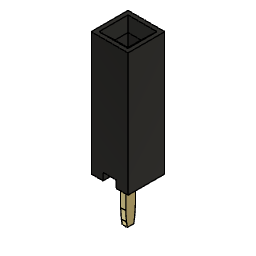
Adjustable_Header_Female (Autodesk Fusion 360 design; units mm, degrees)
Autodesk Fusion 360 part; units mm, degrees
sketch "Sketch1" plane through (0, 0, 0) normal (0, 0, 1) x (1, 0, 0)
  line L0 (1, -1) -> (-1, -1)
  line L1 (-1, -1) -> (-1, 1)
  line L2 (-1, 1) -> (1, 1)
  line L3 (1, 1) -> (1, -1)
  line L4 (1, -1) -> (-1, 1) construction
  line L5 (-1, -1) -> (1, 1) construction
  dimension "d1" = 2
  dimension "d2" = 2
  constraint horizontal L0
  constraint perpendicular L0 L1
  constraint parallel L0 L2
  constraint parallel L1 L3
  constraint coincident L4 origin
  constraint coincident L5 origin
  measures "d1" distance of L1.end L2.end
  measures "d2" distance of L0.end L1.end
extrude "Extrude1" add sketch "Sketch1" along normal blind 8.5 makes body 1
sketch "Sketch2" plane through (0, 0, 8.5) normal (0, 0, 1) x (-1, 0, 0)
  line L0 (-1, -1) -> (1, -1)
  line L1 (1, -1) -> (1, 1)
  line L2 (1, 1) -> (-1, 1)
  line L3 (-1, 1) -> (-1, -1)
  line L4 (-0.45, 0.45) -> (0.45, 0.45)
  line L5 (0.45, 0.45) -> (0.45, -0.45)
  line L6 (0.45, -0.45) -> (-0.45, -0.45)
  line L7 (-0.45, -0.45) -> (-0.45, 0.45)
  line L8 (-0.45, 0.45) -> (0.45, -0.45) construction
  line L9 (0.45, 0.45) -> (-0.45, -0.45) construction
  dimension "d5" = 0.9
  dimension "d6" = 0.9
  constraint horizontal L4
  constraint perpendicular L4 L5
  constraint parallel L4 L6
  constraint parallel L5 L7
  constraint coincident L8 origin
  constraint coincident L9 origin
  measures "d5" distance of L5.end L6.end
  measures "d6" distance of L4.end L5.end
extrude "Extrude2" cut sketch "Sketch2" against normal blind 0.5 contours L4 L5 L6 L7 bodies 1
loft "Loft1" cut profiles "Sketch2" section 1 contours L0 L1 L2 L3 | L4 L5 L6 L7 section 2 face at (0.15, -0.15, 8) on bodies 1 bodies 1
extrude "Extrude3" cut 1 faces at (0.15, -0.15, 8) along direction (0, 0, -1) through all on bodies 1 bodies 1
sketch "Sketch3" plane through (0, 0, 0) normal (0, 0, -1) x (1, 0, 0)
  line L0 (0.45, 0.45) -> (0.45, -0.45)
  line L1 (0.45, -0.45) -> (-0.45, -0.45)
  line L2 (-0.45, -0.45) -> (-0.45, 0.45)
  line L3 (-0.45, 0.45) -> (0.45, 0.45)
  line L4 (-1, -1) -> (1, -1)
  line L5 (1, -1) -> (1, 1)
  line L6 (1, 1) -> (-1, 1)
  line L7 (-1, 1) -> (-1, -1)
  line L8 (0.325, -0.175) -> (-0.325, -0.175)
  line L9 (-0.325, -0.175) -> (-0.325, 0.175)
  line L10 (-0.325, 0.175) -> (0.325, 0.175)
  line L11 (0.325, 0.175) -> (0.325, -0.175)
  line L12 (0.325, -0.175) -> (-0.325, 0.175) construction
  line L13 (-0.325, -0.175) -> (0.325, 0.175) construction
  dimension "d11" = 0.65
  dimension "d12" = 0.35
  constraint horizontal L8
  constraint perpendicular L8 L9
  constraint parallel L8 L10
  constraint parallel L9 L11
  constraint coincident L12 origin
  constraint coincident L13 origin
  measures "d11" distance of L9.end L10.end
  measures "d12" distance of L8.end L9.end
extrude "Extrude4" add sketch "Sketch3" along normal blind 3 separate body contours L8 L9 L10 L11 makes body 2
chamfer "Chamfer1" distance 0.1 distance2 0.7 2 edges at (0.325, 0, -3) (-0.325, 0, -3) measured on face at (0.1083, 0.0583, -3) measured on face at (0.1083, 0.0583, -3) on bodies 2
sketch "Sketch4" plane through (0, 0, 0) normal (0, 0, 1) x (-1, 0, 0)
  line L0 (0.325, 0.175) -> (-0.325, 0.175)
  line L1 (-0.325, 0.175) -> (-0.325, -0.175)
  line L2 (-0.325, -0.175) -> (0.325, -0.175)
  line L3 (0.325, -0.175) -> (0.325, 0.175)
  line L4 (-0.325, 0.175) -> (-0.475, 0.175)
  line L5 (-0.475, 0.175) -> (-0.475, -0.175)
  line L6 (-0.475, -0.175) -> (-0.325, -0.175)
  line L7 (-0.325, -0.175) -> (-0.325, 0.175)
  line L8 (0.325, 0.175) -> (0.475, 0.175)
  line L9 (0.475, 0.175) -> (0.475, -0.175)
  line L10 (0.475, -0.175) -> (0.325, -0.175)
  line L11 (0.325, -0.175) -> (0.325, 0.175)
  dimension "d17" = 0.15
  dimension "d18" = 0.15
  constraint horizontal L4
  constraint vertical L5
  constraint horizontal L6
  constraint vertical L7
  constraint coincident L0.end L1.start
  constraint horizontal L8
  constraint vertical L9
  constraint horizontal L10
  constraint vertical L11
  constraint coincident L0.start L3.end
  measures "d17" distance of L0.end L4.end
  measures "d18" distance of L0.start L8.end
extrude "Extrude5" add sketch "Sketch4" along normal blind 7 contours L3 L8 L9 L10 L11 | L1 L4 L5 L6 L7 bodies 2
extrude "Extrude6" add 1 faces at (0.1083, 0.0583, 0) along direction (0, 0, 1) blind 0.15 on bodies 2 bodies 2
move_body "Move1" bodies 1 2 to x (0, -1, 0) y (1, 0, 0) z (0, 0, 1) at (0, 0, 0)
fillet "Fillet1" radius 5 2 edges at (0, -0.325, -2.3) (0, 0.325, -2.3) on bodies 2
sketch "Sketch5" plane through (0, 0, 0) normal (0, 0, -1) x (1, 0, 0)
  line L0 (-0.45, 0.45) -> (0.45, 0.45)
  line L1 (0.45, 0.45) -> (0.45, -0.45)
  line L2 (0.45, -0.45) -> (-0.45, -0.45)
  line L3 (-0.45, -0.45) -> (-0.45, 0.45)
  line L4 (1, -1) -> (1, 1)
  line L5 (1, 1) -> (-1, 1)
  line L6 (-1, 1) -> (-1, -1)
  line L7 (-1, -1) -> (1, -1)
  line L8 (-0.45, 0.45) -> (0.45, 0.45)
  line L9 (0.45, 0.45) -> (0.45, 1)
  line L10 (0.45, 1) -> (-0.45, 1)
  line L11 (-0.45, 1) -> (-0.45, 0.45)
  line L12 (-0.45, -0.45) -> (0.45, -0.45)
  line L13 (0.45, -0.45) -> (0.45, -1)
  line L14 (0.45, -1) -> (-0.45, -1)
  line L15 (-0.45, -1) -> (-0.45, -0.45)
  constraint horizontal L8
  constraint vertical L9
  constraint horizontal L10
  constraint vertical L11
  constraint coincident L5 L9.end
  constraint coincident L0.start L3.end
  constraint horizontal L12
  constraint vertical L13
  constraint horizontal L14
  constraint vertical L15
  constraint coincident L7 L13.end
  constraint coincident L2.end L3.start
extrude "Extrude7" cut sketch "Sketch5" against normal blind 0.5 contours L0 L5 L8 L9 L10 L11 | L2 L7 L12 L13 L14 L15 bodies 1 2
extrude "Extrude8" add 1 faces at (0.15, 1, 5.8333) along direction (0, 1, 0) blind 0.27 on bodies 1 bodies 1
extrude "Extrude9" add 1 faces at (0.15, -1, 5.8333) along direction (0, -1, 0) blind 0.27 on bodies 1 bodies 1
extrude "Extrude10" add 1 faces at (-1, 0.3333, 2.8333) along direction (-1, 0, 0) blind 0.27 on bodies 1 bodies 1
extrude "Extrude11" add 1 faces at (1, 0.3333, 2.8333) along direction (1, 0, 0) blind 0.27 on bodies 1 bodies 1
pattern_linear "R-Pattern2" count 1 spacing 2.54 along (1, 0, 0) of bodies 2 1 merged
equation "hMWidthNumber = 1"
equation "p = 23455" comment "Bug"
equation "hMNumber_Width = 1" comment "hMWidthNumber bug!***"
equation "hMNumber_Lenght = 1"
equation "d45 = hMNumber_Width"
equation "d46 = hMNumber_Lenght"
